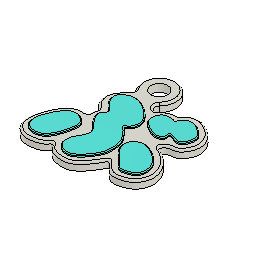
Azusa Keychain v3 (Autodesk Fusion 360 design; units mm, degrees)
Autodesk Fusion 360 part; units mm, degrees
sketch "bu body v1" plane through (0, 0, 0) normal (0, 0, 1) x (1, 0, 0)
  spline S0 degree 5 poles (6, 10.5) (6.065063, 10.484911) (6.192779, 10.453893) (6.377583, 10.405535) (6.613036, 10.338435) (6.897356, 10.247172) (7.179734, 10.142853) (7.465959, 10.020198) (7.757667, 9.877139) (8.050003, 9.718197) (8.334104, 9.552014) (8.600058, 9.388297) (8.839849, 9.234817) (9.049968, 9.094729) (9.235037, 8.96287) (9.405473, 8.828078) (9.572984, 8.677677) (9.746997, 8.501055) (9.930156, 8.294129) (10.119687, 8.058198) (10.309616, 7.797992) (10.492709, 7.519973) (10.662485, 7.23057) (10.815321, 6.934355) (10.949711, 6.634138) (11.065381, 6.331193) (11.162407, 6.025415) (11.240425, 5.715541) (11.297577, 5.39927) (11.330549, 5.073741) (11.335497, 4.736301) (11.308709, 4.385188) (11.247383, 4.020247) (11.150349, 3.643632) (11.018813, 3.260514) (10.855766, 2.878277) (10.66539, 2.505727) (10.452488, 2.152297) (10.221869, 1.827256) (9.977819, 1.53892) (9.723384, 1.293836) (9.460291, 1.096088) (9.189609, 0.946769) (8.912229, 0.84336) (8.629396, 0.779275) (8.343265, 0.743023) (8.057294, 0.718495) (7.775991, 0.688514) (7.504819, 0.638026) (7.249958, 0.557034) (7.018324, 0.444611) (6.816522, 0.308124) (6.648636, 0.158911) (6.515012, 0.009094) (6.409113, -0.132299) (6.321746, -0.261647) (6.248486, -0.381417) (6.198703, -0.502769) (6.190208, -0.638813) (6.234067, -0.78994) (6.328457, -0.939855) (6.466318, -1.070369) (6.641745, -1.175682) (6.852457, -1.265768) (7.097162, -1.35731) (7.374536, -1.468667) (7.681221, -1.612021) (8.011801, -1.79245) (8.359565, -2.010094) (8.717052, -2.261395) (9.076678, -2.540729) (9.431327, -2.841844) (9.774979, -3.15944) (10.103245, -3.490522) (10.412998, -3.833844) (10.702073, -4.189493) (10.968943, -4.558418) (11.212402, -4.941989) (11.431241, -5.341529) (11.623953, -5.757892) (11.788346, -6.190936) (11.921586, -6.639432) (12.020495, -7.10122) (12.08177, -7.573292) (12.102236, -8.051907) (12.079078, -8.532685) (12.010094, -9.010715) (11.89393, -9.480658) (11.73032, -9.936851) (11.520068, -10.373587) (11.265023, -10.785386) (10.968068, -11.167274) (10.633088, -11.515054) (10.264971, -11.825595) (9.869557, -12.097074) (9.453675, -12.329332) (9.024961, -12.523866) (8.591258, -12.683074) (8.160115, -12.809652) (7.738244, -12.90594) (7.330981, -12.973272) (6.94178, -13.011369) (6.57162, -13.017607) (6.218656, -12.986641) (5.87954, -12.912463) (5.550532, -12.790143) (5.22875, -12.617789) (4.91323, -12.398197) (4.606381, -12.141169) (4.314242, -11.863739) (4.044143, -11.585721) (3.80297, -11.326395) (3.59503, -11.100386) (3.420448, -10.914683) (3.272467, -10.763222) (3.138377, -10.629684) (3.005218, -10.501181) (2.86425, -10.37912) (2.716044, -10.291525) (2.565668, -10.274848) (2.417355, -10.353647) (2.270333, -10.52514) (2.121152, -10.770776) (1.96516, -11.064232) (1.798474, -11.381585) (1.619239, -11.708118) (1.426962, -12.03549) (1.222143, -12.360416) (1.00579, -12.682751) (0.778981, -13.00384) (0.542406, -13.324726) (0.295931, -13.644498) (0.038798, -13.96071) (-0.230213, -14.269733) (-0.512603, -14.567129) (-0.80998, -14.848015) (-1.123887, -15.107431) (-1.45562, -15.340721) (-1.806073, -15.543821) (-2.175613, -15.713365) (-2.563945, -15.846848) (-2.969984, -15.942746) (-3.391723, -16.000681) (-3.826112, -16.021528) (-4.268893, -16.007632) (-4.714728, -15.96244) (-5.157425, -15.889962) (-5.590117, -15.79429) (-6.005485, -15.679102) (-6.395919, -15.54713) (-6.753797, -15.399759) (-7.071478, -15.236262) (-7.342696, -15.054924) (-7.564397, -14.854897) (-7.738676, -14.637957) (-7.874143, -14.409992) (-7.988841, -14.183373) (-8.107024, -13.975807) (-8.248902, -13.805556) (-8.424099, -13.688075) (-8.619463, -13.631098) (-8.806468, -13.63452) (-8.959875, -13.693408) (-9.078015, -13.800501) (-9.185247, -13.947561) (-9.313207, -14.124919) (-9.485005, -14.321319) (-9.707468, -14.524332) (-9.977617, -14.721817) (-10.285449, -14.903153) (-10.618041, -15.060446) (-10.963541, -15.190045) (-11.313643, -15.292894) (-11.662625, -15.372672) (-12.007181, -15.434465) (-12.345937, -15.483155) (-12.679092, -15.522084) (-13.008024, -15.551215) (-13.334842, -15.567116) (-13.661869, -15.564499) (-13.991141, -15.537324) (-14.323904, -15.480063) (-14.660095, -15.388953) (-14.997896, -15.263084) (-15.334146, -15.103536) (-15.664682, -14.912671) (-15.984708, -14.69336) (-16.289149, -14.448251) (-16.573016, -14.179) (-16.831758, -13.885559) (-17.061334, -13.566717) (-17.258292, -13.220601) (-17.419854, -12.845173) (-17.54399, -12.43876) (-17.629497, -12.000517) (-17.676099, -11.531029) (-17.684401, -11.032419) (-17.655699, -10.50804) (-17.591832, -9.962289) (-17.495016, -9.40037) (-17.367684, -8.828079) (-17.212329, -8.251581) (-17.031338, -7.677184) (-16.826844, -7.111127) (-16.600529, -6.559337) (-16.353723, -6.02735) (-16.087595, -5.52028) (-15.803313, -5.042779) (-15.502219, -4.598993) (-15.185999, -4.192526) (-14.856854, -3.826398) (-14.517666, -3.503005) (-14.172172, -3.224079) (-13.825145, -2.99065) (-13.481932, -2.80285) (-13.147956, -2.659701) (-12.828235, -2.558917) (-12.526881, -2.496691) (-12.24664, -2.467506) (-11.988332, -2.463879) (-11.751536, -2.476941) (-11.535519, -2.497088) (-11.339905, -2.514685) (-11.165871, -2.520532) (-11.013975, -2.508034) (-10.881364, -2.475588) (-10.75873, -2.429394) (-10.63949, -2.374584) (-10.53669, -2.299513) (-10.477572, -2.179388) (-10.471078, -2.002666) (-10.493213, -1.783319) (-10.509601, -1.545348) (-10.491069, -1.312274) (-10.435204, -1.0926) (-10.360105, -0.883324) (-10.292362, -0.677158) (-10.256777, -0.468639) (-10.265906, -0.260319) (-10.323256, -0.058178) (-10.425645, 0.131996) (-10.566087, 0.309467) (-10.735591, 0.479057) (-10.924436, 0.648726) (-11.123457, 0.828092) (-11.325661, 1.026376) (-11.526129, 1.251506) (-11.720864, 1.509822) (-11.905901, 1.805582) (-12.076433, 2.140591) (-12.225633, 2.513667) (-12.34467, 2.920606) (-12.424294, 3.354794) (-12.456049, 3.807659) (-12.433601, 4.269191) (-12.354106, 4.728421) (-12.219351, 5.173949) (-12.037501, 5.594371) (-11.822733, 5.979041) (-11.59205, 6.319277) (-11.362823, 6.609439) (-11.149972, 6.848106) (-10.963457, 7.039096) (-10.805268, 7.192844) (-10.667728, 7.326685) (-10.538902, 7.457891) (-10.406883, 7.598573) (-10.265054, 7.747713) (-10.113661, 7.896246) (-9.959699, 8.036172) (-9.856962, 8.180042) (-9.8, 8.3) (-9.745047, 8.489958) (-9.72783, 8.731004) (-9.73174, 8.956407) (-9.84407, 9.218534) (-9.981308, 9.474361) (-10.124097, 9.710727) (-10.244739, 9.921678) (-10.335604, 10.077581) (-10.392721, 10.197265) (-10.42488, 10.275805) (-10.437264, 10.308112) knots 0 0 0 0 0 0 0.00286533 0.00573066 0.00859599 0.01146132 0.01432665 0.01719198 0.02005731 0.02292264 0.02578797 0.0286533 0.03151862 0.03438395 0.03724928 0.04011461 0.04297994 0.04584527 0.0487106 0.05157593 0.05444126 0.05730659 0.06017192 0.06303725 0.06590258 0.06876791 0.07163324 0.07449857 0.0773639 0.08022923 0.08309456 0.08595989 0.08882521 0.09169054 0.09455587 0.0974212 0.10028653 0.10315186 0.10601719 0.10888252 0.11174785 0.11461318 0.11747851 0.12034384 0.12320917 0.1260745 0.12893983 0.13180516 0.13467049 0.13753582 0.14040115 0.14326648 0.14613181 0.14899713 0.15186246 0.15472779 0.15759312 0.16045845 0.16332378 0.16618911 0.16905444 0.17191977 0.1747851 0.17765043 0.18051576 0.18338109 0.18624642 0.18911175 0.19197708 0.19484241 0.19770774 0.20057307 0.2034384 0.20630372 0.20916905 0.21203438 0.21489971 0.21776504 0.22063037 0.2234957 0.22636103 0.22922636 0.23209169 0.23495702 0.23782235 0.24068768 0.24355301 0.24641834 0.24928367 0.252149 0.25501433 0.25787966 0.26074499 0.26361032 0.26647564 0.26934097 0.2722063 0.27507163 0.27793696 0.28080229 0.28366762 0.28653295 0.28939828 0.29226361 0.29512894 0.29799427 0.3008596 0.30372493 0.30659026 0.30945559 0.31232092 0.31518625 0.31805158 0.32091691 0.32378223 0.32664756 0.32951289 0.33237822 0.33524355 0.33810888 0.34097421 0.34383954 0.34670487 0.3495702 0.35243553 0.35530086 0.35816619 0.36103152 0.36389685 0.36676218 0.36962751 0.37249284 0.37535817 0.3782235 0.38108883 0.38395415 0.38681948 0.38968481 0.39255014 0.39541547 0.3982808 0.40114613 0.40401146 0.40687679 0.40974212 0.41260745 0.41547278 0.41833811 0.42120344 0.42406877 0.4269341 0.42979943 0.43266476 0.43553009 0.43839542 0.44126074 0.44412607 0.4469914 0.44985673 0.45272206 0.45558739 0.45845272 0.46131805 0.46418338 0.46704871 0.46991404 0.47277937 0.4756447 0.47851003 0.48137536 0.48424069 0.48710602 0.48997135 0.49283668 0.49570201 0.49856734 0.50143266 0.50429799 0.50716332 0.51002865 0.51289398 0.51575931 0.51862464 0.52148997 0.5243553 0.52722063 0.53008596 0.53295129 0.53581662 0.53868195 0.54154728 0.54441261 0.54727794 0.55014327 0.5530086 0.55587393 0.55873926 0.56160458 0.56446991 0.56733524 0.57020057 0.5730659 0.57593123 0.57879656 0.58166189 0.58452722 0.58739255 0.59025788 0.59312321 0.59598854 0.59885387 0.6017192 0.60458453 0.60744986 0.61031519 0.61318052 0.61604585 0.61891117 0.6217765 0.62464183 0.62750716 0.63037249 0.63323782 0.63610315 0.63896848 0.64183381 0.64469914 0.64756447 0.6504298 0.65329513 0.65616046 0.65902579 0.66189112 0.66475645 0.66762178 0.67048711 0.67335244 0.67621777 0.67908309 0.68194842 0.68481375 0.68767908 0.69054441 0.69340974 0.69627507 0.6991404 0.70200573 0.70487106 0.70773639 0.71060172 0.71346705 0.71633238 0.71919771 0.72206304 0.72492837 0.7277937 0.73065903 0.73352436 0.73638968 0.73925501 0.74212034 0.74498567 0.747851 0.75071633 0.75358166 0.75644699 0.75931232 0.76217765 0.76504298 0.76790831 0.77077364 0.77363897 0.7765043 0.77936963 0.78223496 0.78510029 0.78796562 0.79083095 0.79369628 0.79563186 0.79563186 0.79563186 0.79563186 0.79563186 0.79563186
  spline S1 degree 5 poles (-3.37025, 9.02762) (-3.381026, 9.015832) (-3.413807, 8.979699) (-3.469142, 8.916504) (-3.551235, 8.811616) (-3.65, 8.65) (-3.695123, 8.421671) (-3.720726, 8.17981) (-3.678824, 7.904382) (-3.565485, 7.618229) (-3.386109, 7.349092) (-3.155724, 7.122965) (-2.89818, 6.957537) (-2.647145, 6.853882) (-2.435964, 6.802226) (-2.28504, 6.791093) (-2.189885, 6.815375) (-2.109322, 6.884631) (-1.997864, 7.008618) (-1.838195, 7.182842) (-1.63282, 7.393019) (-1.394519, 7.620076) (-1.138053, 7.844608) (-0.869351, 8.05243) (-0.585586, 8.235337) (-0.281111, 8.389251) (0.048383, 8.513177) (0.40102, 8.607828) (0.764088, 8.674368) (1.109543, 8.713185) (1.405115, 8.726789) (1.626033, 8.723058) (1.764976, 8.717555) (1.846459, 8.738149) (1.926296, 8.821718) (2.051715, 8.987667) (2.245138, 9.228445) (2.512431, 9.520098) (2.846069, 9.828421) (3.230426, 10.117143) (3.645897, 10.354604) (4.074151, 10.522645) (4.500435, 10.618381) (4.913154, 10.649055) (5.304179, 10.628751) (5.59592, 10.585231) (5.802404, 10.544429) (5.934938, 10.51509) (6, 10.5) knots 0.87538872 0.87538872 0.87538872 0.87538872 0.87538872 0.87538872 0.87679083 0.87965616 0.88252149 0.88538682 0.88825215 0.89111748 0.89398281 0.89684814 0.89971347 0.9025788 0.90544413 0.90830946 0.91117479 0.91404011 0.91690544 0.91977077 0.9226361 0.92550143 0.92836676 0.93123209 0.93409742 0.93696275 0.93982808 0.94269341 0.94555874 0.94842407 0.9512894 0.95415473 0.95702006 0.95988539 0.96275072 0.96561605 0.96848138 0.9713467 0.97421203 0.97707736 0.97994269 0.98280802 0.98567335 0.98853868 0.99140401 0.99426934 0.99713467 1 1 1 1 1 1
  arc A0 (-3.37025, 9.02762) -> (-10.244891, 9.921604) centre (-6.47401, 12.039654) ccw
  circle A1 centre (-6.47401, 12.039654) radius 2.156841
  point P0 (-10.437264, 10.308112)
  constraint concentric A0 A1
extrude "Extrude1" add sketch "bu body v1" along normal blind 2 contours S0 S1 A0 picked at (-0.585522, -4.397233)
fillet "Fillet1" radius 0.5 3 edges at (-5.916279, 16.328548, 2) (-2.558101, -15.834484, 2) (-0.504534, 8.270126, 2)
sketch "bu middle v1" plane through (0, 0, 2) normal (0, 0, 1) x (1, 0, 0)
  spline S0 degree 5 poles (-1.4999, -2.061475) (-1.452072, -2.10212) (-1.322, -2.230573) (-1.043975, -2.548135) (-0.677775, -2.969646) (-0.281745, -3.449201) (0.082894, -3.937293) (0.376754, -4.399455) (0.589411, -4.822257) (0.728607, -5.206356) (0.814294, -5.563021) (0.870443, -5.909119) (0.918446, -6.263053) (0.968261, -6.639579) (1.017009, -7.048039) (1.053881, -7.493409) (1.063229, -7.97657) (1.028513, -8.494887) (0.93562, -9.042667) (0.777073, -9.611644) (0.553759, -10.191537) (0.272494, -10.770792) (-0.055478, -11.33728) (-0.41637, -11.879018) (-0.795556, -12.384869) (-1.179377, -12.845268) (-1.556846, -13.252909) (-1.921545, -13.603516) (-2.272994, -13.896367) (-2.614603, -14.133183) (-2.952045, -14.317215) (-3.291392, -14.452209) (-3.637505, -14.541531) (-3.991961, -14.586977) (-4.352409, -14.588548) (-4.714053, -14.545606) (-5.070669, -14.457767) (-5.415717, -14.325776) (-5.743637, -14.152682) (-6.050261, -13.94382) (-6.332075, -13.705281) (-6.585724, -13.44267) (-6.807517, -13.159947) (-6.992696, -12.857751) (-7.135628, -12.533632) (-7.231388, -12.185113) (-7.27711, -11.812304) (-7.273221, -11.420224) (-7.225235, -11.022392) (-7.14346, -10.639759) (-7.039987, -10.293687) (-6.926184, -9.999926) (-6.810356, -9.763221) (-6.694435, -9.569134) (-6.574583, -9.3869) (-6.445791, -9.183572) (-6.305454, -8.9353) (-6.15723, -8.639292) (-6.009364, -8.306666) (-5.873228, -7.95584) (-5.761789, -7.606105) (-5.688092, -7.270198) (-5.663778, -6.95025) (-5.697785, -6.64236) (-5.794942, -6.339627) (-5.954758, -6.03557) (-6.169715, -5.727939) (-6.427073, -5.417891) (-6.711405, -5.108076) (-7.006976, -4.801028) (-7.299978, -4.497601) (-7.58133, -4.194966) (-7.847549, -3.886197) (-8.097545, -3.563222) (-8.330393, -3.218973) (-8.54247, -2.850038) (-8.72544, -2.458688) (-8.86241, -2.056212) (-8.931894, -1.66066) (-8.915809, -1.291596) (-8.806816, -0.96551) (-8.614639, -0.691532) (-8.376038, -0.465598) (-8.149435, -0.271336) (-7.995991, -0.086773) (-7.966091, 0.111019) (-8.080011, 0.339535) (-8.326704, 0.609114) (-8.675062, 0.924306) (-9.081556, 1.284348) (-9.499388, 1.684007) (-9.886925, 2.114265) (-10.216616, 2.563061) (-10.472839, 3.016672) (-10.649601, 3.461141) (-10.748305, 3.883639) (-10.775453, 4.273951) (-10.740478, 4.6257) (-10.65327, 4.9382) (-10.522908, 5.215765) (-10.357191, 5.465135) (-10.161995, 5.693552) (-9.940586, 5.906366) (-9.693301, 6.105432) (-9.418706, 6.28986) (-9.114534, 6.45639) (-8.778652, 6.599936) (-8.410162, 6.714005) (-8.009632, 6.791415) (-7.578884, 6.825123) (-7.120923, 6.809002) (-6.639811, 6.738673) (-6.140562, 6.612259) (-5.629034, 6.431293) (-5.111755, 6.200088) (-4.595735, 5.924928) (-4.088285, 5.613325) (-3.596838, 5.273257) (-3.128762, 4.912395) (-2.691177, 4.537374) (-2.29078, 4.152943) (-1.933649, 3.761507) (-1.625011, 3.36421) (-1.36902, 2.961801) (-1.168522, 2.55554) (-1.024832, 2.148183) (-0.937502, 1.744719) (-0.904093, 1.35375) (-0.919976, 0.986014) (-0.978272, 0.651406) (-1.069561, 0.356216) (-1.139855, 0.132321) (-1.25, -0.1) (-1.32199, -0.226753) (-1.45, -0.45) (-1.6, -0.6) (-1.777393, -0.780508) (-1.954611, -0.937272) (-2.215996, -1.079186) (-2.388363, -1.167136) (-2.380394, -1.319241) (-2.16808, -1.542544) (-1.8622, -1.772999) (-1.7, -1.9) (-1.557894, -2.013719) (-1.4999, -2.061475) knots 0 0 0 0 0 0 0.0070922 0.0141844 0.0212766 0.02836879 0.03546099 0.04255319 0.04964539 0.05673759 0.06382979 0.07092199 0.07801418 0.08510638 0.09219858 0.09929078 0.10638298 0.11347518 0.12056738 0.12765957 0.13475177 0.14184397 0.14893617 0.15602837 0.16312057 0.17021277 0.17730496 0.18439716 0.19148936 0.19858156 0.20567376 0.21276596 0.21985816 0.22695035 0.23404255 0.24113475 0.24822695 0.25531915 0.26241135 0.26950355 0.27659574 0.28368794 0.29078014 0.29787234 0.30496454 0.31205674 0.31914894 0.32624113 0.33333333 0.34042553 0.34751773 0.35460993 0.36170213 0.36879433 0.37588652 0.38297872 0.39007092 0.39716312 0.40425532 0.41134752 0.41843972 0.42553191 0.43262411 0.43971631 0.44680851 0.45390071 0.46099291 0.46808511 0.4751773 0.4822695 0.4893617 0.4964539 0.5035461 0.5106383 0.5177305 0.5248227 0.53191489 0.53900709 0.54609929 0.55319149 0.56028369 0.56737589 0.57446809 0.58156028 0.58865248 0.59574468 0.60283688 0.60992908 0.61702128 0.62411348 0.63120567 0.63829787 0.64539007 0.65248227 0.65957447 0.66666667 0.67375887 0.68085106 0.68794326 0.69503546 0.70212766 0.70921986 0.71631206 0.72340426 0.73049645 0.73758865 0.74468085 0.75177305 0.75886525 0.76595745 0.77304965 0.78014184 0.78723404 0.79432624 0.80141844 0.80851064 0.81560284 0.82269504 0.82978723 0.83687943 0.84397163 0.85106383 0.85815603 0.86524823 0.87234043 0.87943262 0.88652482 0.89361702 0.90070922 0.90780142 0.91489362 0.92198582 0.92907801 0.93617021 0.94326241 0.95035461 0.95744681 0.96453901 0.97163121 0.9787234 0.9858156 0.9929078 1 1 1 1 1 1
extrude "Extrude2" add sketch "bu middle v1" along normal blind 0.5 contours S0 picked at (-4.110013, 0.939885)
fillet "Fillet2" radius 0.22 1 edges at (-7.970461, -3.722493, 2.5)
sketch "bu left" plane through (0, 0, 2) normal (0, 0, 1) x (1, 0, 0)
  spline S0 degree 5 poles (-11.231861, -4.270515) (-11.336824, -4.247043) (-11.545933, -4.210112) (-11.855201, -4.185908) (-12.252947, -4.218486) (-12.718916, -4.365109) (-13.152383, -4.609525) (-13.555625, -4.93999) (-13.932303, -5.343655) (-14.286299, -5.807679) (-14.620914, -6.319834) (-14.937918, -6.869322) (-15.236727, -7.447403) (-15.513346, -8.048375) (-15.760638, -8.668458) (-15.968956, -9.304163) (-16.126601, -9.950777) (-16.220429, -10.600932) (-16.236208, -11.242803) (-16.159638, -11.859481) (-15.979038, -12.431684) (-15.687883, -12.939919) (-15.287155, -13.366718) (-14.788417, -13.699201) (-14.21463, -13.930389) (-13.595036, -14.057196) (-12.961076, -14.078997) (-12.342125, -13.996103) (-11.760814, -13.807996) (-11.230016, -13.512591) (-10.755492, -13.10897) (-10.337549, -12.599549) (-9.973056, -11.992447) (-9.657308, -11.303875) (-9.38591, -10.560305) (-9.155557, -9.793896) (-8.964881, -9.038162) (-8.815253, -8.32361) (-8.711659, -7.673276) (-8.663444, -7.098532) (-8.685425, -6.594055) (-8.793663, -6.144469) (-9.000404, -5.732506) (-9.309913, -5.345802) (-9.712434, -4.986228) (-10.186031, -4.668749) (-10.59952, -4.465275) (-10.916151, -4.350946) (-11.126897, -4.293988) (-11.231861, -4.270515) knots 0 0 0 0 0 0 0.02222222 0.04444444 0.06666667 0.08888889 0.11111111 0.13333333 0.15555556 0.17777778 0.2 0.22222222 0.24444444 0.26666667 0.28888889 0.31111111 0.33333333 0.35555556 0.37777778 0.4 0.42222222 0.44444444 0.46666667 0.48888889 0.51111111 0.53333333 0.55555556 0.57777778 0.6 0.62222222 0.64444444 0.66666667 0.68888889 0.71111111 0.73333333 0.75555556 0.77777778 0.8 0.82222222 0.84444444 0.86666667 0.88888889 0.91111111 0.93333333 0.95555556 0.97777778 1 1 1 1 1 1
extrude "Extrude3" add sketch "bu left" along normal blind 0.5 contours S0 picked at (-10.904147, -5.686433)
fillet "Fillet3" radius 0.22 1 edges at (-13.901072, -13.980707, 2.5)
sketch "bu right v1" plane through (0, 0, 2) normal (0, 0, 1) x (1, 0, 0)
  spline S0 degree 5 poles (1.67024, -3.758478) (1.716223, -3.688448) (1.814622, -3.551379) (1.980446, -3.355283) (2.232333, -3.115127) (2.581135, -2.856607) (2.94721, -2.645865) (3.318096, -2.48846) (3.690017, -2.388896) (4.069391, -2.350214) (4.467388, -2.373874) (4.895728, -2.459561) (5.362289, -2.605046) (5.866016, -2.805939) (6.39799, -3.056111) (6.944124, -3.348284) (7.487262, -3.674556) (8.009585, -4.026964) (8.494731, -4.397997) (8.93042, -4.781205) (9.309384, -5.171504) (9.628465, -5.565154) (9.88819, -5.959831) (10.092177, -6.354665) (10.24658, -6.750273) (10.359654, -7.148874) (10.439275, -7.553257) (10.490058, -7.965565) (10.510882, -8.386211) (10.491616, -8.812595) (10.412046, -9.238313) (10.249367, -9.65431) (9.984677, -10.049749) (9.609292, -10.412966) (9.132533, -10.732432) (8.584365, -10.997585) (8.005656, -11.199381) (7.441113, -11.33088) (6.930809, -11.387855) (6.545962, -11.368425) (6.228912, -11.28516) (5.943888, -11.131439) (5.729871, -10.938034) (5.521707, -10.679241) (5.3, -10.4) (5.027655, -10.063768) (4.756057, -9.752857) (4.449678, -9.442919) (4.112176, -9.136774) (3.751357, -8.831287) (3.377914, -8.519842) (3.004242, -8.194323) (2.643207, -7.84733) (2.306982, -7.474185) (2.005729, -7.075313) (1.747849, -6.655205) (1.540407, -6.221016) (1.389533, -5.781241) (1.300728, -5.344474) (1.279477, -4.917855) (1.330459, -4.506944) (1.430776, -4.194595) (1.538719, -3.971563) (1.624256, -3.828509) (1.67024, -3.758478) knots 0 0 0 0 0 0 0.01666667 0.03333333 0.05 0.06666667 0.08333333 0.1 0.11666667 0.13333333 0.15 0.16666667 0.18333333 0.2 0.21666667 0.23333333 0.25 0.26666667 0.28333333 0.3 0.31666667 0.33333333 0.35 0.36666667 0.38333333 0.4 0.41666667 0.43333333 0.45 0.46666667 0.48333333 0.5 0.51666667 0.53333333 0.55 0.56666667 0.58333333 0.6 0.61666667 0.63333333 0.65 0.66666667 0.68333333 0.7 0.71666667 0.73333333 0.75 0.76666667 0.78333333 0.8 0.81666667 0.83333333 0.85 0.86666667 0.88333333 0.9 0.91666667 0.93333333 0.95 0.96666667 0.98333333 1 1 1 1 1 1
extrude "Extrude5" add sketch "bu right v1" along normal blind 0.5 contours S0 picked at (8.015818, -9.45374)
fillet "Fillet5" radius 0.22 1 edges at (9.957153, -10.041695, 2.5)
sketch "bu top v1" plane through (0, 0, 2) normal (0, 0, 1) x (1, 0, 0)
  spline S0 degree 5 poles (-0.376362, 2.822844) (-0.328442, 2.769384) (-0.228286, 2.663685) (-0.065526, 2.508668) (0.174398, 2.308739) (0.505389, 2.070329) (0.859308, 1.844525) (1.227609, 1.633166) (1.602049, 1.438711) (1.975318, 1.264101) (2.341833, 1.112653) (2.697952, 0.987871) (3.041395, 0.893136) (3.370857, 0.831435) (3.685552, 0.80506) (3.98477, 0.815359) (4.267468, 0.862352) (4.531677, 0.944932) (4.773778, 1.06146) (4.987827, 1.210236) (5.164848, 1.39003) (5.29214, 1.600577) (5.359045, 1.83993) (5.363173, 2.101552) (5.315689, 2.371936) (5.248976, 2.626898) (5.206991, 2.837488) (5.231962, 2.977936) (5.352194, 3.032979) (5.569792, 3.005227) (5.868651, 2.910282) (6.222224, 2.772039) (6.600825, 2.618139) (6.980439, 2.474838) (7.345463, 2.364295) (7.686176, 2.303945) (7.997702, 2.305311) (8.278349, 2.372984) (8.528261, 2.503664) (8.747816, 2.684794) (8.937747, 2.898521) (9.099464, 3.126443) (9.235246, 3.353772) (9.348621, 3.574434) (9.444283, 3.793666) (9.526496, 4.022146) (9.597712, 4.271417) (9.65718, 4.548971) (9.699353, 4.853029) (9.715768, 5.175066) (9.697168, 5.502953) (9.63562, 5.823979) (9.526438, 6.127684) (9.370719, 6.409376) (9.174237, 6.669572) (8.945162, 6.912093) (8.692086, 7.142573) (8.422086, 7.36686) (8.138399, 7.589322) (7.839444, 7.81165) (7.521203, 8.032992) (7.178973, 8.249814) (6.808586, 8.443331) (6.4, 8.6) (6, 8.7) (5.496202, 8.776193) (5.1, 8.75) (4.8, 8.7) (4.5, 8.6) (4.15, 8.4) (3.9, 8.2) (3.7, 8) (3.45, 7.69) (3.3, 7.45) (3.125898, 7.135388) (2.973886, 6.579446) (3.231932, 6.587617) (2.75, 6.75) (2.5, 6.85) (2.3, 6.9) (2.1, 6.95) (1.823161, 6.983625) (1.6, 7) (1.337702, 7.009475) (1.130946, 7.007317) (0.923032, 6.982793) (0.710069, 6.936741) (0.489985, 6.868739) (0.264201, 6.774998) (0.037673, 6.648711) (-0.182652, 6.482802) (-0.388943, 6.272008) (-0.573778, 6.015265) (-0.731322, 5.717862) (-0.857007, 5.389418) (-0.947264, 5.042024) (-0.999214, 4.688252) (-1.010423, 4.339382) (-0.978527, 4.003148) (-0.901279, 3.683132) (-0.777083, 3.380136) (-0.63974, 3.150452) (-0.515809, 2.984445) (-0.424283, 2.876304) (-0.376362, 2.822844) knots 0 0 0 0 0 0 0.01 0.02 0.03 0.04 0.05 0.06 0.07 0.08 0.09 0.1 0.11 0.12 0.13 0.14 0.15 0.16 0.17 0.18 0.19 0.2 0.21 0.22 0.23 0.24 0.25 0.26 0.27 0.28 0.29 0.3 0.31 0.32 0.33 0.34 0.35 0.36 0.37 0.38 0.39 0.4 0.41 0.42 0.43 0.44 0.45 0.46 0.47 0.48 0.49 0.5 0.51 0.52 0.53 0.54 0.55 0.56 0.57 0.58 0.59 0.6 0.61 0.62 0.63 0.64 0.65 0.66 0.67 0.68 0.69 0.7 0.71 0.72 0.73 0.74 0.75 0.76 0.77 0.78 0.79 0.8 0.81 0.82 0.83 0.84 0.85 0.86 0.87 0.88 0.89 0.9 0.91 0.92 0.93 0.94 0.95 0.96 0.97 0.98 0.99 1 1 1 1 1 1
extrude "Extrude6" add sketch "bu top v1" along normal blind 0.5 contours S0 picked at (5.261328, 5.939147)
fillet "Fillet6" radius 0.22 1 edges at (9.514843, 6.122224, 2.5)
